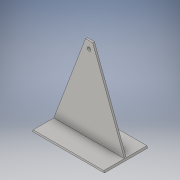
# Autodesk Inventor part: PitchingMachineSupport
Saved by Autodesk Inventor 2016 SP1 (Build 200210100, 210)
## iProperties
Created: 2016-01-12
Part Number: PitchingMachineSupport
Material: Generic
Document SubType Name: Modeling
Designer: steele
Density: 1 g/cm^3
Appearance: Default
Author: steele
Autodesk Inventor part; units mm, degrees
ref_plane "YZ Plane" through (0, 0, 0) normal (1, 0, 0) x (0, 1, 0)
ref_plane "XZ Plane" through (0, 0, 0) normal (0, 1, 0) x (-1, 0, 0)
ref_plane "XY Plane" through (0, 0, 0) normal (0, 0, 1) x (1, 0, 0)
sketch "Sketch1" plane through (0, 0, 0) normal (0, 0, 1) x (1, 0, 0)
  line L0 (0, 0) -> (127, 0)
  line L1 (127, 0) -> (12.7, 304.8)
  line L2 (12.7, 304.8) -> (0, 304.8)
  line L3 (0, 304.8) -> (0, 0) construction
  line L4 (0, 0) -> (-127, 0)
  line L5 (-127, 0) -> (-12.7, 304.8)
  line L6 (-12.7, 304.8) -> (0, 304.8)
  circle A0 centre (0, 279.4) radius 6.35
  dimension "d0" = 304.8
  dimension "d1" = 254
  dimension "d2" = 25.4
  dimension "d3" = 12.7
  dimension "d4" = 279.4
  constraints: 14 end point, 2 symmetric about line, 1 centre point, 1 horizontal, 1 parallel, 1 point on line, 1 vertical
  measures "d0" distance between parallel lines of L0 L2
  measures "d1" distance of L0.end L5.start
  measures "d2" distance of L1.end L6.start
  measures "d3" diameter of A0
  measures "d4" distance of A0.centre L0.start
extrude "Extrusion1" add sketch "Sketch1" along normal mid plane 6.35
sketch "Sketch2" plane through (0, 0, 0) normal (0, 0, 1) x (1, 0, 0)
  line L0 (-127, 0) -> (127, 0) projected
  line L1 (-127, 0) -> (127, 0)
  line L2 (127, 0) -> (124.6187, 6.35)
  line L3 (127, 0) -> (12.7, 304.8) projected
  line L4 (-12.7, 304.8) -> (-127, 0) projected
  line L5 (-124.6187, 6.35) -> (-127, 0)
  line L6 (-124.6187, 6.35) -> (124.6187, 6.35)
  point P0 (0, 0)
  dimension "d7" = 6.35
  constraints: 8 end point, 2 collinear, 2 point on line, 1 horizontal
  measures "d7" distance between parallel lines of L6 L0
extrude "Extrusion2" add sketch "Sketch2" along normal mid plane 152.4
equation "\"d0\" = pitchingMachineltSideHeight"
equation "\"d1\" = pitchingMachineSideWidth"
equation "\"d2\" = pitchingMachineltTopWidth"
equation "\"d3\" = pitchingMachineSideHoleDiam"
equation "\"d4\" = pitchingMachineSideHoleHeight"
equation "\"d5\" = pitchingMachineSideDepth"
equation "\"d7\" = pitchingMachineSideDepth"
equation "\"d8\" = pitchingMachineltSupportWidth"
equation "\"pitchingMachineltSideHeight\" = 304.8"
equation "\"pitchingMachineSideWidth\" = 254"
equation "\"pitchingMachineSideDepth\" = 6.35"
equation "\"pitchingMachineSideHoleDiam\" = 12.7"
equation "\"pitchingMachineltTopWidth\" = 25.4"
equation "\"pitchingMachineltSupportWidth\" = 152.4"
equation "\"pitchingMachineSideHoleHeight\" = 279.4"
body "Solid1"
